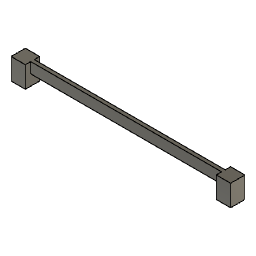
Top of Stand v6 (Autodesk Fusion 360 design; units mm, degrees)
Autodesk Fusion 360 part; units mm, degrees
sketch "Sketch1" plane through (0, 0, 0) normal (0, 0, 1) x (1, 0, 0)
  line L0 (68.9309, 100) -> (378.9309, 100)
  line L1 (378.9309, 100) -> (378.9309, 79.8)
  line L2 (378.9309, 79.8) -> (68.9309, 79.8)
  line L3 (68.9309, 79.8) -> (68.9309, 100)
  line L4 (73.9309, 95) -> (84.1309, 95)
  line L5 (84.1309, 95) -> (84.1309, 84.8)
  line L6 (84.1309, 84.8) -> (73.9309, 84.8)
  line L7 (73.9309, 84.8) -> (73.9309, 95)
  line L8 (89.1309, 100) -> (89.1309, 79.8)
  line L9 (363.7309, 95) -> (373.9309, 95)
  line L10 (373.9309, 95) -> (373.9309, 84.8)
  line L11 (373.9309, 84.8) -> (363.7309, 84.8)
  line L12 (363.7309, 84.8) -> (363.7309, 95)
  line L13 (358.7309, 100) -> (358.7309, 79.8)
  line L14 (89.1309, 92.4) -> (358.7309, 92.4)
  line L15 (358.7309, 92.4) -> (358.7309, 87.4)
  line L16 (358.7309, 87.4) -> (89.1309, 87.4)
  line L17 (89.1309, 87.4) -> (89.1309, 92.4)
  dimension "d1" = 310
  dimension "d2" = 20.2
  dimension "d3" = 20.2
  dimension "d4" = 5
  dimension "d5" = 5
  dimension "d6" = 5
  dimension "d7" = 5
  dimension "d8" = 20.2
  dimension "d9" = 20.2
  dimension "d10" = 5
  dimension "d11" = 5
  dimension "d12" = 5
  dimension "d13" = 5
  dimension "d14" = 5
  dimension "d15" = 7.6
  dimension "d16" = 7.6
  constraint horizontal L0
  constraint vertical L1
  constraint horizontal L2
  constraint vertical L3
  constraint horizontal L4
  constraint vertical L5
  constraint horizontal L6
  constraint vertical L7
  constraint coincident L0 L8.start
  constraint coincident L2 L8.end
  constraint perpendicular L2 L8
  constraint horizontal L9
  constraint vertical L10
  constraint horizontal L11
  constraint vertical L12
  constraint coincident L0 L13.start
  constraint coincident L2 L13.end
  constraint perpendicular L2 L13
  constraint horizontal L14
  constraint vertical L15
  constraint horizontal L16
  constraint vertical L17
  constraint coincident L13 L15.end
  constraint coincident L8 L14.start
  measures "d1" distance of L1 L3
  measures "d2" distance of L0.start L2.end
  measures "d3" distance of L3 L8
  measures "d4" distance of L5 L8
  measures "d5" distance of L0 L4
  measures "d6" distance of L3 L7
  measures "d7" distance of L2 L6
  measures "d8" distance of L0.end L1.end
  measures "d9" distance of L1 L13
  measures "d10" distance of L0 L9
  measures "d11" distance of L1 L10
  measures "d12" distance of L2 L11
  measures "d13" distance of L12 L13
  measures "d14" distance of L14 L16
  measures "d15" distance of L0 L14
  measures "d16" distance of L2 L16
extrude "Extrude1" add sketch "Sketch1" against normal blind 2.5 contours L4 L5 L6 L7 | L9 L10 L11 L12 makes body 1 at (367.1309, 91.6, 0) makes body 2 at (77.3309, 91.6, 0)
extrude "Extrude2" add sketch "Sketch1" against normal blind 30 contours L0 L2 L3 L8 L17 | L0 L1 L2 L13 L15 bodies 1 2
extrude "Extrude3" add sketch "Sketch1" against normal blind 15 contours L8 L13 L14 L15 L16 L17 bodies 1 2
